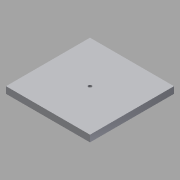
# Autodesk Inventor part: Plate
Saved by Autodesk Inventor 2013 (Build 170138000, 138)
## iProperties
Created: 2013-01-18
Part Number: Plate
Material: Aluminum 6061
Document SubType Name: Modeling
Designer: Naphat
Density: 1 g/cm^3
Author: Naphat
Autodesk Inventor part; units mm, degrees
ref_plane "YZ Plane" through (0, 0, 0) normal (1, 0, 0) x (0, 1, 0)
ref_plane "XZ Plane" through (0, 0, 0) normal (0, 1, 0) x (-1, 0, 0)
ref_plane "XY Plane" through (0, 0, 0) normal (0, 0, 1) x (1, 0, 0)
sketch "Sketch1" plane through (0, 0, 0) normal (0, 1, 0) x (-1, 0, 0)
  line L0 (-54.3339, 60.0501) -> (-54.3339, -193.9499)
  line L1 (-54.3339, -193.9499) -> (199.6661, -193.9499)
  line L2 (199.6661, -193.9499) -> (199.6661, 60.0501)
  line L3 (199.6661, 60.0501) -> (-54.3339, 60.0501)
  point P0 (0, 0)
  dimension "d0" = 254
  dimension "d1" = 254
  constraints: 8 end point, 2 perpendicular, 1 parallel, 1 vertical
  measures "d0" distance of L0.start L0.end
  measures "d1" distance of L0.end L1.end
extrude "Extrusion1" add sketch "Sketch1" along normal blind 20
sketch "Sketch2" plane through (0, 20, 0) normal (0, 1, 0) x (1, 0, 0)
  line L0 (54.3339, -60.0501) -> (54.3339, 193.9499) projected
  line L1 (-199.6661, 193.9499) -> (54.3339, -60.0501) construction
  line L2 (-199.6661, -60.0501) -> (54.3339, 193.9499) construction
  circle A0 centre (-72.6661, 66.9499) radius 5
  point P0 (0, 0)
  dimension "d4" = 10
  constraints: 4 end point, 2 midpoint, 1 centre point, 1 perpendicular, 1 point on line
  measures "d4" diameter of A0
extrude "Extrusion2" cut sketch "Sketch2" against normal blind 25.4
body "Solid1"
